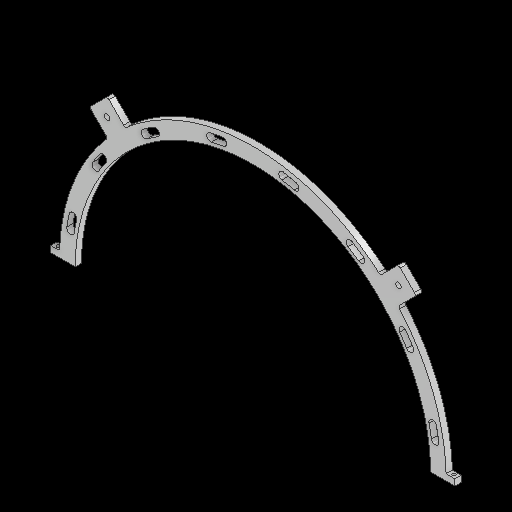
# Autodesk Inventor part: half_ring_1
Saved by Autodesk Inventor 2026.1 (Build 301233000, 233)
## iProperties
Created: 2025-09-17
Part Number: half_ring_1
Material: Aluminum 6061
Document SubType Name: Modeling
Designer: drago
Density: 2.7 g/cm^3
Appearance: Aluminum - Polished
Mass: 433.666 g
Surface Area: 584.563 cm^2
Volume: 160.617 cm^3
Author: drago
Autodesk Inventor part; units mm, degrees
ref_plane "YZ Plane" through (0, 0, 0) normal (1, 0, 0) x (0, 1, 0)
ref_plane "XZ Plane" through (0, 0, 0) normal (0, 1, 0) x (-1, 0, 0)
ref_plane "XY Plane" through (0, 0, 0) normal (0, 0, 1) x (1, 0, 0)
sketch "Sketch7" plane through (0, 0, 0) normal (0, 0, 1) x (1, 0, 0)
  circle A0 centre (-231.5775, 231.5775) radius 4.25
  line L0 (-231.5775, 203.2932) -> (-203.2932, 231.5775)
  line L1 (-203.2932, 231.5775) -> (-231.5775, 259.8617)
  line L2 (-231.5775, 259.8617) -> (-259.8617, 231.5775)
  line L3 (-259.8617, 231.5775) -> (-231.5775, 203.2932)
  line L4 (-231.5775, 203.2932) -> (-231.5775, 259.8617) construction
  line L5 (-203.2932, 231.5775) -> (-259.8617, 231.5775) construction
  line L6 (-231.5775, 203.2932) -> (-191.5775, 203.2932) construction
  arc A1 (289.9795, 47.2262) -> (285.9788, 67.3391) centre (0, 0) ccw construction
  arc A2 (295.9015, 48.1906) -> (291.8191, 68.7143) centre (0, 0) ccw
  arc A3 (284.0576, 46.2617) -> (280.1386, 65.9639) centre (0, 0) ccw
  arc A4 (284.0576, 46.2617) -> (295.9015, 48.1906) centre (289.9795, 47.2262) ccw
  arc A5 (291.8191, 68.7143) -> (280.1386, 65.9639) centre (285.9788, 67.3391) ccw
  line L7 (0, 0) -> (289.9795, 47.2262) construction
  line L8 (0, 0) -> (293.8, 0) construction
  line L9 (0, 0) -> (285.9788, 67.3391) construction
  circle A6 centre (0, 0) radius 307.5
  circle A7 centre (0, 0) radius 282.5
  line L10 (-203.2932, 231.5775) -> (-185.1143, 213.3986)
  line L11 (-231.5775, 203.2932) -> (-213.3986, 185.1143)
  line L12 (-307.5, 0) -> (0, 0)
  line L13 (0, 0) -> (307.5, 0)
  line L14 (-231.5775, -203.2932) -> (-259.8617, -231.5775)
  line L15 (-259.8617, -231.5775) -> (-231.5775, -259.8617)
  circle A8 centre (-231.5775, -231.5775) radius 4.25
  line L16 (-231.5775, -259.8617) -> (-203.2932, -231.5775)
  line L17 (-203.2932, -231.5775) -> (-231.5775, -203.2932)
  line L18 (-203.2932, -231.5775) -> (-185.1143, -213.3986)
  line L19 (-231.5775, -203.2932) -> (-213.3986, -185.1143)
  line L20 (203.2932, -231.5775) -> (231.5775, -259.8617)
  line L21 (231.5775, -259.8617) -> (259.8617, -231.5775)
  circle A9 centre (231.5775, -231.5775) radius 4.25
  line L22 (259.8617, -231.5775) -> (231.5775, -203.2932)
  line L23 (231.5775, -203.2932) -> (203.2932, -231.5775)
  line L24 (231.5775, -203.2932) -> (213.3986, -185.1143)
  line L25 (203.2932, -231.5775) -> (185.1143, -213.3986)
  line L26 (231.5775, 203.2932) -> (259.8617, 231.5775)
  line L27 (259.8617, 231.5775) -> (231.5775, 259.8617)
  circle A10 centre (231.5775, 231.5775) radius 4.25
  line L28 (231.5775, 259.8617) -> (203.2932, 231.5775)
  line L29 (203.2932, 231.5775) -> (231.5775, 203.2932)
  line L30 (203.2932, 231.5775) -> (185.1143, 213.3986)
  line L31 (231.5775, 203.2932) -> (213.3986, 185.1143)
  arc A11 (254.9356, 157.7589) -> (243.3099, 175.158) centre (0, 0) ccw
  arc A12 (243.3099, 175.158) -> (233.571, 168.1471) centre (238.4404, 171.6526) ccw
  arc A13 (244.7314, 151.4444) -> (233.571, 168.1471) centre (0, 0) ccw
  arc A14 (244.7314, 151.4444) -> (254.9356, 157.7589) centre (249.8335, 154.6017) ccw
  arc A15 (175.158, 243.3099) -> (157.7589, 254.9356) centre (0, 0) ccw
  arc A16 (157.7589, 254.9356) -> (151.4444, 244.7314) centre (154.6017, 249.8335) ccw
  arc A17 (168.1471, 233.571) -> (151.4444, 244.7314) centre (0, 0) ccw
  arc A18 (168.1471, 233.571) -> (175.158, 243.3099) centre (171.6526, 238.4404) ccw
  arc A19 (68.7143, 291.8191) -> (48.1906, 295.9015) centre (0, 0) ccw
  arc A20 (48.1906, 295.9015) -> (46.2617, 284.0576) centre (47.2262, 289.9795) ccw
  arc A21 (65.9639, 280.1386) -> (46.2617, 284.0576) centre (0, 0) ccw
  arc A22 (65.9639, 280.1386) -> (68.7143, 291.8191) centre (67.3391, 285.9788) ccw
  arc A23 (-48.1906, 295.9015) -> (-68.7143, 291.8191) centre (0, 0) ccw
  arc A24 (-68.7143, 291.8191) -> (-65.9639, 280.1386) centre (-67.3391, 285.9788) ccw
  arc A25 (-46.2617, 284.0576) -> (-65.9639, 280.1386) centre (0, 0) ccw
  arc A26 (-46.2617, 284.0576) -> (-48.1906, 295.9015) centre (-47.2262, 289.9795) ccw
  arc A27 (-157.7589, 254.9356) -> (-175.158, 243.3099) centre (0, 0) ccw
  arc A28 (-175.158, 243.3099) -> (-168.1471, 233.571) centre (-171.6526, 238.4404) ccw
  arc A29 (-151.4444, 244.7314) -> (-168.1471, 233.571) centre (0, 0) ccw
  arc A30 (-151.4444, 244.7314) -> (-157.7589, 254.9356) centre (-154.6017, 249.8335) ccw
  arc A31 (-243.3099, 175.158) -> (-254.9356, 157.7589) centre (0, 0) ccw
  arc A32 (-254.9356, 157.7589) -> (-244.7314, 151.4444) centre (-249.8335, 154.6017) ccw
  arc A33 (-233.571, 168.1471) -> (-244.7314, 151.4444) centre (0, 0) ccw
  arc A34 (-233.571, 168.1471) -> (-243.3099, 175.158) centre (-238.4404, 171.6526) ccw
  arc A35 (-291.8191, 68.7143) -> (-295.9015, 48.1906) centre (0, 0) ccw
  arc A36 (-295.9015, 48.1906) -> (-284.0576, 46.2617) centre (-289.9795, 47.2262) ccw
  arc A37 (-280.1386, 65.9639) -> (-284.0576, 46.2617) centre (0, 0) ccw
  arc A38 (-280.1386, 65.9639) -> (-291.8191, 68.7143) centre (-285.9788, 67.3391) ccw
  arc A39 (-295.9015, -48.1906) -> (-291.8191, -68.7143) centre (0, 0) ccw
  arc A40 (-291.8191, -68.7143) -> (-280.1386, -65.9639) centre (-285.9788, -67.3391) ccw
  arc A41 (-284.0576, -46.2617) -> (-280.1386, -65.9639) centre (0, 0) ccw
  arc A42 (-284.0576, -46.2617) -> (-295.9015, -48.1906) centre (-289.9795, -47.2262) ccw
  arc A43 (-254.9356, -157.7589) -> (-243.3099, -175.158) centre (0, 0) ccw
  arc A44 (-243.3099, -175.158) -> (-233.571, -168.1471) centre (-238.4404, -171.6526) ccw
  arc A45 (-244.7314, -151.4444) -> (-233.571, -168.1471) centre (0, 0) ccw
  arc A46 (-244.7314, -151.4444) -> (-254.9356, -157.7589) centre (-249.8335, -154.6017) ccw
  arc A47 (-175.158, -243.3099) -> (-157.7589, -254.9356) centre (0, 0) ccw
  arc A48 (-157.7589, -254.9356) -> (-151.4444, -244.7314) centre (-154.6017, -249.8335) ccw
  arc A49 (-168.1471, -233.571) -> (-151.4444, -244.7314) centre (0, 0) ccw
  arc A50 (-168.1471, -233.571) -> (-175.158, -243.3099) centre (-171.6526, -238.4404) ccw
  arc A51 (-68.7143, -291.8191) -> (-48.1906, -295.9015) centre (0, 0) ccw
  arc A52 (-48.1906, -295.9015) -> (-46.2617, -284.0576) centre (-47.2262, -289.9795) ccw
  arc A53 (-65.9639, -280.1386) -> (-46.2617, -284.0576) centre (0, 0) ccw
  arc A54 (-65.9639, -280.1386) -> (-68.7143, -291.8191) centre (-67.3391, -285.9788) ccw
  arc A55 (48.1906, -295.9015) -> (68.7143, -291.8191) centre (0, 0) ccw
  arc A56 (68.7143, -291.8191) -> (65.9639, -280.1386) centre (67.3391, -285.9788) ccw
  arc A57 (46.2617, -284.0576) -> (65.9639, -280.1386) centre (0, 0) ccw
  arc A58 (46.2617, -284.0576) -> (48.1906, -295.9015) centre (47.2262, -289.9795) ccw
  arc A59 (157.7589, -254.9356) -> (175.158, -243.3099) centre (0, 0) ccw
  arc A60 (175.158, -243.3099) -> (168.1471, -233.571) centre (171.6526, -238.4404) ccw
  arc A61 (151.4444, -244.7314) -> (168.1471, -233.571) centre (0, 0) ccw
  arc A62 (151.4444, -244.7314) -> (157.7589, -254.9356) centre (154.6017, -249.8335) ccw
  arc A63 (243.3099, -175.158) -> (254.9356, -157.7589) centre (0, 0) ccw
  arc A64 (254.9356, -157.7589) -> (244.7314, -151.4444) centre (249.8335, -154.6017) ccw
  arc A65 (233.571, -168.1471) -> (244.7314, -151.4444) centre (0, 0) ccw
  arc A66 (233.571, -168.1471) -> (243.3099, -175.158) centre (238.4404, -171.6526) ccw
  arc A67 (291.8191, -68.7143) -> (295.9015, -48.1906) centre (0, 0) ccw
  arc A68 (295.9015, -48.1906) -> (284.0576, -46.2617) centre (289.9795, -47.2262) ccw
  arc A69 (280.1386, -65.9639) -> (284.0576, -46.2617) centre (0, 0) ccw
  arc A70 (280.1386, -65.9639) -> (291.8191, -68.7143) centre (285.9788, -67.3391) ccw
  point P0 (-202.8328, 231.1171)
  point P1 (-231.1171, 202.8328)
  point P2 (-282.5, 0)
  point P3 (282.5, 0)
  point P4 (231.1171, 202.8328)
  point P5 (202.8328, 231.1171)
  dimension "d131" = 8.5
  dimension "d132" = 231.5775
  dimension "d133" = 231.5775
  dimension "d135" = 45
  dimension "d137" = 40
  dimension "d138" = 40
  dimension "d144" = 293.8
  dimension "d145" = 9.25
  dimension "d146" = 4
  dimension "d147" = 12
  dimension "d148" = 615
  dimension "d149" = 565
  dimension "d152" = 360
  dimension "d156" = 360
  constraints: 134 point on circle, 71 centre point, 64 end point, 9 point on line, 6 coincident, 4 tangent, 3 horizontal, 2 equal length, 2 midpoint, 2 parallel, 1 perpendicular, 235 other
  measures "d131" diameter of A0
  measures "d132" horizontal distance of point (0, 0) A0.centre
  measures "d133" horizontal distance of point (0, 0) A0.centre
  measures "d135" angle of L6 L0
  measures "d137" distance of L1.end L2.end
  measures "d138" distance between parallel lines of L2 L0
  measures "d144" radius of A1
  measures "d145" angle of L8 L7
  measures "d146" angle of L7 L9
  measures "d147" diameter of A5
  measures "d148" diameter of A6
  measures "d149" diameter of A7
extrude "Extrusion11" add sketch "Sketch7" against normal blind 10 contours L3 L2 L1 L0 | L0 A6 L11 | L0 L10 A6 | A6 L10 A7 L11 | L11 A7 L12 A6 | A6 L30 A7 L10 | L30 L29 A6 | A6 L31 A7 L30 | L29 L31 A6 | L29 L28 L27 L26 | A6 L13 A7 L31
sketch "Sketch8" plane through (-307.5, 0, 0) normal (0, -1, 0) x (1, 0, 0)
  line L0 (25, 0) -> (590, 0) projected
  line L1 (25, 0) -> (-14, 0)
  line L2 (-14, 0) -> (-14, -10)
  line L3 (-14, -10) -> (25, -10)
  line L4 (25, -10) -> (25, 0)
  circle A0 centre (-7, -5) radius 2.6
  line L5 (590, 0) -> (629, 0)
  line L6 (629, 0) -> (629, -10)
  line L7 (629, -10) -> (590, -10)
  line L8 (590, -10) -> (590, 0)
  circle A1 centre (622, -5) radius 2.6
  dimension "d160" = 39
  dimension "d161" = 10
  dimension "d162" = 5.2
  dimension "d163" = 5
  dimension "d164" = 7
  dimension "d165" = 39
  dimension "d166" = 10
  dimension "d167" = 5.2
  dimension "d168" = 7
  dimension "d169" = 5
  constraints: 16 end point, 4 parallel, 2 centre point, 2 horizontal, 2 perpendicular
  measures "d160" distance of L3.end L2.end
  measures "d161" distance of L1.end L2.end
  measures "d162" diameter of A0
  measures "d163" distance from line of L1 A0.centre
  measures "d164" distance from line of L2 A0.centre
  measures "d165" distance of L6.end L7.end
  measures "d166" distance of L5.end L6.end
  measures "d167" diameter of A1
  measures "d168" distance from line of L6 A1.centre
  measures "d169" distance from line of L7 A1.centre
extrude "Extrusion12" add sketch "Sketch8" against normal blind 10 contours L4 L3 L2 L1 | A0 | L5 L6 L7 L8 | A1
fillet "Fillet4" radius 4 8 edges at (-231.1171, 202.8328, -5) (-259.8617, 231.5775, -5) (-202.8328, 231.1171, -5) (-231.5775, 259.8617, -5) (231.5775, 259.8617, -5) (259.8617, 231.5775, -5) (202.8328, 231.1171, -5) (231.1171, 202.8328, -5)
hole "Hole6" at (-314.5, 0, -5) at (314.5, 0, -5) direction (0, 1, 0) diameter 5.2 end through all
equation "\"bar_screw_hole_diam\" = 8.5"
equation "\"foot_length\" = 14"
equation "\"tube_rim_diam\" = 605"
equation "\"tube_inner_diam\" = 541"
equation "\"tube_outer_diam\" = 561"
equation "\"ring_delta\" = 2"
equation "\"bar_delta\" = 5"
equation "\"bar_circle_diam\" = 655"
equation "\"ring_inner_diam\" = 565"
equation "\"ring_outer_diam\" = 615"
equation "\"slot_angle\" = 9.25deg"
equation "\"slot_diam\" = 12"
equation "\"slots_circle_diam\" = 587.6"
equation "\"foot_screw_diam\" = 5.2"
equation "\"bar_fillet\" = 4"
body "Solid2"
